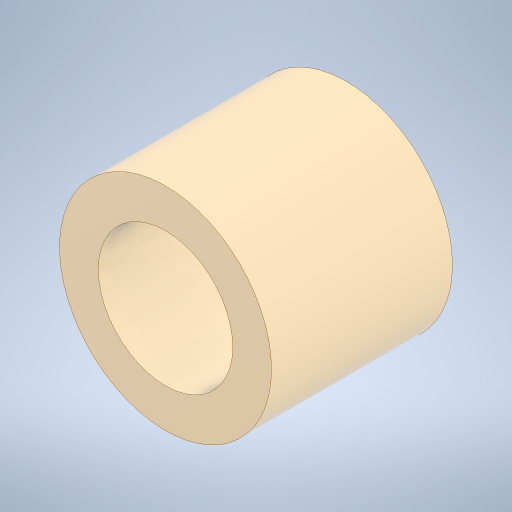
# Autodesk Inventor part: TutupShaftRodaDepan
Saved by Autodesk Inventor 2024 (Build 280153000, 153)
## iProperties
Created: 2025-12-11
Part Number: TutupShaftRodaDepan
Material: Generic
Document SubType Name: Modeling
Designer: risda
Density: 1 g/cm^3
Appearance: Smooth - Off-White
Author: risda
Autodesk Inventor part; units mm, degrees
ref_plane "YZ Plane" through (0, 0, 0) normal (1, 0, 0) x (0, 1, 0)
ref_plane "XZ Plane" through (0, 0, 0) normal (0, 1, 0) x (-1, 0, 0)
ref_plane "XY Plane" through (0, 0, 0) normal (0, 0, 1) x (1, 0, 0)
sketch "Sketch1" plane through (0, 0, 0) normal (0, 0, 1) x (1, 0, 0)
  circle A0 centre (0, 0) radius 2.6
  circle A1 centre (0, 0) radius 4.1
  dimension "d0" = 5.2
  dimension "d1" = 8.2
  constraints: 2 centre point, 2 coincident
  measures "d0" diameter of A0
  measures "d1" diameter of A1
extrude "Extrusion1" add sketch "Sketch1" along normal blind 0.5 contours A0
extrude "Extrusion2" add sketch "Sketch1" along normal blind 7
body "Solid1"
